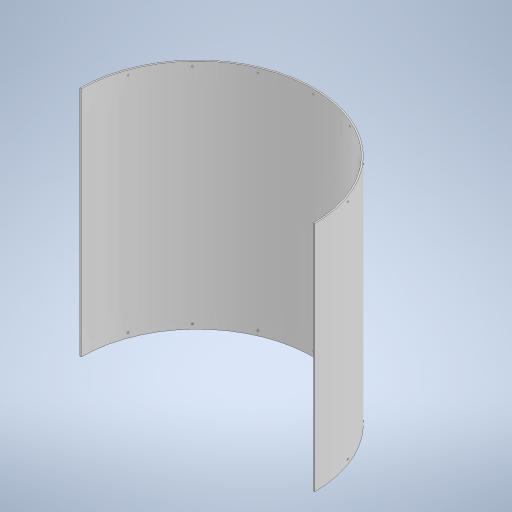
# Autodesk Inventor part: Aspa
Saved by Autodesk Inventor 2024 (Build 280153000, 153)
## iProperties
Created: 2024-04-25
Part Number: Aspa
Material: Genérico
Document SubType Name: Modeling
Designer: alexa
Density: 1 g/cm^3
Appearance: Valor por defecto
Author: alexa
Autodesk Inventor part; units mm, degrees
note: some values were not read from the file. Chosen so that the rebuilt part matches the saved one: pattern direction of "Circular Pattern2".
ref_plane "YZ Plane" through (0, 0, 0) normal (1, 0, 0) x (0, 1, 0)
sketch "Sketch2" plane through (0, 0, 0) normal (1, 0, 0) x (0, 1, 0)
  line L0 (0, 0) -> (121.8561, 0)
  line L1 (3, -250) -> (497, -250)
  line L2 (500, -250) -> (500, -253)
  line L3 (500, -253) -> (0, -253)
  line L4 (0, -253) -> (0, -250)
  line L5 (500, 0) -> (497, 0)
  line L6 (3, -250) -> (0, -250)
  line L7 (497, -250) -> (500, -250)
  point P0 (3, 0)
  dimension "d7" = 500
  constraints: 16 end point, 5 horizontal, 2 parallel, 1 perpendicular, 1 point on line
  measures "d7" distance of L2.end L3.end
revolve "Revolution1" add sketch "Sketch2" angle 180 mid plane about axis through (0, 0, 0) along (0, 1, 0)
ref_plane "Work Plane2" through (0, 0, -253) normal (0, 0, 1) x (1, 0, 0)
sketch "Sketch5" plane through (0, 0, -253) normal (0, 0, 1) x (1, 0, 0)
  line L0 (250, 500) -> (-250, 500) projected
  circle A0 centre (0, 490) radius 1.5
  point P0 (0, 0)
  dimension "d24" = 3
  constraints: 1 centre point
  measures "d24" diameter of A0
extrude "Extrusion3" cut sketch "Sketch5" along normal blind 5
ref_plane "Work Plane3" through (0, 250, 0) normal (0, 1, 0) x (1, 0, 0)
mirror "Mirror1" about plane through (0, 250, 0) normal (0, 1, 0) of "Extrusion3"
pattern_circular "Circular Pattern2" count 7 over 140 about axis through (0, -10, 0) along (0, 1, 0) of "Extrusion3", "Mirror1" both ways yes
body "Solid2"
